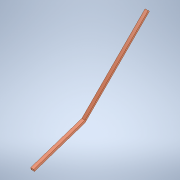
# Autodesk Inventor part: side1
Saved by Autodesk Inventor 2021.1 (Build 251245000, 245)
## iProperties
Created: 2020-09-07
Part Number: side1
Material: Wood (Walnut)
Document SubType Name: Modeling
Designer: robst
Density: 0.55 g/cm^3
Appearance: Walnut - Natural Polished
Author: robst
Autodesk Inventor part; units mm, degrees
ref_plane "YZ Plane" through (0, 0, 0) normal (1, 0, 0) x (0, 1, 0)
ref_plane "XZ Plane" through (0, 0, 0) normal (0, 1, 0) x (-1, 0, 0)
ref_plane "XY Plane" through (0, 0, 0) normal (0, 0, 1) x (1, 0, 0)
sketch "Sketch1" plane through (0, 0, 0) normal (1, 0, 0) x (0, 1, 0)
  line L0 (0, 0) -> (2155.2615, -2155.2615)
  line L1 (0, 0) -> (3048, 0) construction
  line L2 (2155.2615, -2155.2615) -> (2119.3404, -2191.1825)
  line L3 (2119.3404, -2191.1825) -> (0, -71.842)
  line L4 (0, -71.842) -> (0, 0)
  line L5 (2119.3404, -2191.1825) -> (1688.2882, -2622.2348)
  line L6 (1688.2882, -2622.2348) -> (1652.3671, -2586.3138)
  line L7 (1652.3671, -2586.3138) -> (1645.6913, -2579.6379)
  line L8 (1645.6913, -2579.6379) -> (2076.7436, -2148.5856)
  line L9 (0, 0) -> (-508, 1524)
  line L10 (-508, 1524) -> (-441.7397, 1546.0868)
  line L11 (-441.7397, 1546.0868) -> (110.4339, -110.4339)
  line L12 (0, 0) -> (35.921, -107.7631)
  dimension "d0" = 3048
  dimension "d1" = 45
  dimension "d2" = 50.8
  dimension "d3" = 609.6
  dimension "d4" = 50.8
  dimension "d5" = 508
  dimension "d6" = 1524
  constraints: 26 end point, 4 perpendicular, 4 point on line, 3 parallel, 1 equal length, 1 horizontal, 1 vertical
  measures "d0" distance of L0.start L0.end
  measures "d1" angle of L0 L1
  measures "d2" distance of L0.end L2.end
  measures "d3" distance of L2.end L5.end
  measures "d4" distance of L5.end L6.end
  measures "d5" horizontal distance of L9.end L0.start
  measures "d6" vertical distance of L9.end L0.start
extrude "Extrusion2" add sketch "Sketch1" along normal blind 101.6 contours L9 L10 L11 L0 | L0 L2 L3 L12
body "Solid2"
